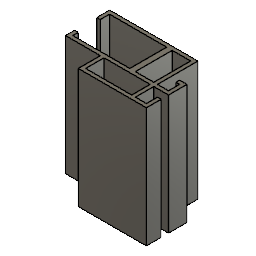
Upper Clip v3 (Autodesk Fusion 360 design; units mm, degrees)
Autodesk Fusion 360 part; units mm, degrees
sketch "Sketch1" plane through (0, 0, 0) normal (0, 1, 0) x (1, 0, 0)
  line L0 (0, 0) -> (0, -4)
  line L1 (0, -4) -> (2, -4)
  line L2 (2, -4) -> (2, 0)
  line L3 (2, 0) -> (0, 0)
  line L4 (2, -4) -> (33, -4)
  line L5 (33, -4) -> (33, 16)
  line L6 (33, 16) -> (0, 16)
  line L7 (0, 16) -> (0, 12)
  line L8 (0, 12) -> (2, 12)
  line L9 (2, 12) -> (2, 15)
  line L10 (2, 15) -> (33, 15)
  line L11 (33, -4) -> (33, -3)
  line L12 (2, -3) -> (33, -3)
  line L13 (33, -4) -> (34.000001, -4)
  line L14 (34.000001, -4) -> (36.000001, -4)
  line L15 (36.000001, -4) -> (36.000001, 16)
  line L16 (36.000001, 16) -> (33, 16)
  line L17 (36.000001, -4) -> (36.000001, -5)
  line L18 (36.000001, -5) -> (0, -5)
  line L19 (0, -5) -> (0, -4)
  line L20 (33, 16) -> (33, 18)
  line L21 (33, 18) -> (48, 18.000001)
  line L22 (48, 18.000001) -> (48.000001, 5.000001)
  line L23 (48.000001, 5.000001) -> (46.000001, 5.000001)
  line L24 (46.000001, 5.000001) -> (46, 16.000001)
  line L25 (46, 16.000001) -> (36.000001, 16)
  line L26 (36.000001, -5) -> (56.000001, -5)
  line L27 (56.000001, -5) -> (56.000001, 5)
  line L28 (56.000001, 5) -> (52.000001, 5)
  line L29 (52.000001, 5) -> (52.000001, 3)
  line L30 (52.000001, 3) -> (54.000001, 3)
  line L31 (54.000001, 3) -> (54.000001, -3)
  line L32 (54.000001, -3) -> (36.000001, -3)
  dimension "d1" = 4
  dimension "d2" = 31
  dimension "d3" = 20
  dimension "d4" = 33
  dimension "d5" = 2
  dimension "d6" = 3
  dimension "d7" = 2
  dimension "d8" = 2
  dimension "d9" = 15
  dimension "d10" = 13
  dimension "d11" = 2
  dimension "d12" = 11
  dimension "d13" = 20
  constraint coincident L0.start L3.end
  constraint perpendicular L0 L1
  constraint perpendicular L1 L2
  constraint perpendicular L0 L3
  constraint perpendicular L6 L7
  constraint coincident L5 L10.end
  constraint perpendicular L5 L10
  constraint coincident L5 L11.end
  constraint perpendicular L4 L11
  constraint coincident L2 L12.start
  constraint perpendicular L5 L12
  constraint perpendicular L11 L13
  constraint perpendicular L14 L15
  constraint perpendicular L14 L17
  constraint perpendicular L17 L18
  constraint perpendicular L1 L19
  constraint parallel L16 L25
  constraint perpendicular L26 L27
  constraint perpendicular L27 L28
  constraint perpendicular L26 L29
  constraint perpendicular L27 L30
  constraint perpendicular L30 L31
  constraint perpendicular L15 L32
  measures "d1" distance of L0.start L0.end
  measures "d2" distance of L1.end L4.end
  measures "d3" distance of L4.end L5.end
  measures "d4" distance of L5.end L6.end
  measures "d5" distance of L7.end L8.end
  measures "d6" distance of L8.end L9.end
  measures "d8" distance of L5.end L20.end
extrude "Extrude1" add sketch "Sketch1" along normal blind 65
move_face "OffsetFaces1" offset 1 1 faces at (22, 21.666667, -16)
extrude "Extrude2" cut 1 faces at (12.333333, 21.666667, -15) along direction (0, 0, -1) blind 1
extrude "Extrude3" add 1 faces at (38, 21.666667, -18) along direction (-0.00000008, 0, -1) blind 5
extrude "Extrude4" cut 1 faces at (42.666667, 43.333333, -16.000001) along direction (-0.00000008, 0, -1) blind 5
extrude "Extrude5" add 1 faces at (47.333334, 43.333333, -5.000001) along direction (0.00000008, 0, 1) blind 8
delete_face "DeleteFace1" 1 faces at (36.000001, 21.666667, -3.333333)
sketch "Sketch2" plane through (0, 0, 0) normal (0, 1, 0) x (1, 0, 0)
sketch "Sketch3" plane through (0, 0, 0) normal (0, 1, 0) x (1, 0, 0)
  line L0 (0, -5) -> (56.000001, -5)
  line L1 (48.000001, -5) -> (48.000001, -17)
  line L2 (48.000001, -17) -> (19.000001, -17)
  line L3 (19.000001, -17) -> (19.000001, -5)
  line L4 (21, -5) -> (21, -15)
  line L5 (21, -15) -> (46.000001, -15)
  line L6 (46.000001, -15) -> (46.000001, -5)
  dimension "d25" = 12
  dimension "d26" = 29
  constraint perpendicular L0 L3
  constraint coincident L0 L4.start
  constraint perpendicular L0 L4
  constraint perpendicular L4 L5
  constraint perpendicular L0 L6
extrude "Extrude6" add sketch "Sketch3" along normal blind 65 contours L0 L1 L2 L3 L4 L5 L6 picked at (37.666667, -16.333333)
extrude "Extrude7" cut 1 faces at (42.666666, 43.333333, -21.000001) along direction (-0.00000008, 0, -1) blind 1
extrude "Extrude8" add 1 faces at (37.999999, 21.666667, -23) along direction (-0.00000008, 0, -1) blind 1
sketch "Sketch4" plane through (0, 0, 0) normal (0, 1, 0) x (1, 0, 0)
  line L0 (48.000001, -17) -> (56.000001, -17)
  line L1 (56.000001, -17) -> (56.000001, -9)
  line L2 (56.000001, -9) -> (54.000001, -9)
  line L3 (54.000001, -9) -> (54.000001, -15)
  line L4 (48.000001, -17) -> (48.000001, -5)
  line L5 (54.000001, -15) -> (48.000001, -15)
  point P0 (48.000001, -17)
  dimension "d33" = 8
  constraint horizontal L0
  constraint perpendicular L1 L2
  constraint perpendicular L0 L3
  constraint perpendicular L3 L5
extrude "Extrude9" add sketch "Sketch4" along normal blind 65
extrude "Extrude10" add 1 faces at (11, 43.333333, -17) along direction (0, 0, -1) blind 2
extrude "Extrude11" cut 1 faces at (12.333333, 21.666667, -16) along direction (0, 0, -1) blind 2
sketch "Sketch5" plane through (0, 0, 0) normal (0, 1, 0) x (1, 0, 0)
extrude "Extrude12" add 1 faces at (42.666666, 43.333333, -22.000001) along direction (0.00000008, 0, 1) blind 5
extrude "Extrude13" cut 1 faces at (37.999999, 21.666667, -24) along direction (0.00000008, 0, 1) blind 5
delete_face "DeleteFace2" 1 faces at (38, 43.333333, -19)
extrude "Extrude14" add 1 faces at (12.333333, 21.666667, -18) along direction (0, 0, 1) blind 1
